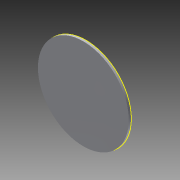
# Autodesk Inventor part: basis
Saved by Autodesk Inventor 2014 (Build 180170000, 170)
## iProperties
Created: 2015-03-19
Part Number: basis
Material: ABS Plastic
Document SubType Name: Modeling
Designer: MSI
Density: 1 g/cm^3
Appearance: Smooth - White
Author: MSI
Autodesk Inventor part; units mm, degrees
ref_plane "YZ Plane" through (0, 0, 0) normal (1, 0, 0) x (0, 1, 0)
ref_plane "XZ Plane" through (0, 0, 0) normal (0, 1, 0) x (-1, 0, 0)
ref_plane "XY Plane" through (0, 0, 0) normal (0, 0, 1) x (1, 0, 0)
sketch "Sketch1" plane through (0, 0, 0) normal (0, 1, 0) x (-1, 0, 0)
  circle A0 centre (0, 0) radius 77.5
  dimension "d0" = 155
  constraints: 1 centre point, 1 coincident
  measures "d0" diameter of A0
extrude "Extrusion1" add sketch "Sketch1" along normal blind 2
sketch "Sketch2" plane through (0, 2, 0) normal (0, 1, 0) x (1, 0, 0)
  circle A0 centre (0, 0) radius 77.5 projected
  line L0 (0, 0) -> (0, 77.5) construction
  line L1 (0, 0) -> (3.3805, 77.4262) construction
  line L2 (0, 0) -> (-3.3805, 77.4262) construction
  line L3 (0, 0) -> (-67.117, 38.75) construction
  line L4 (0, 0) -> (-65.3628, 41.6407) construction
  line L5 (0, 0) -> (-68.7433, 35.7855) construction
  line L6 (0, 0) -> (-67.117, -38.75) construction
  line L7 (0, 0) -> (-68.7433, -35.7855) construction
  line L8 (0, 0) -> (-65.3628, -41.6407) construction
  line L9 (0, 0) -> (0, -77.5) construction
  line L10 (0, 0) -> (-3.3805, -77.4262) construction
  line L11 (0, 0) -> (3.3805, -77.4262) construction
  line L12 (0, 0) -> (67.117, -38.75) construction
  line L13 (0, 0) -> (65.3628, -41.6407) construction
  line L14 (0, 0) -> (68.7433, -35.7855) construction
  line L15 (0, 0) -> (67.117, 38.75) construction
  line L16 (0, 0) -> (68.7433, 35.7855) construction
  line L17 (0, 0) -> (65.3628, 41.6407) construction
  arc A1 (46.2658, -18.96) -> (46.2658, 18.96) centre (0, 0) ccw
  arc A2 (6.7131, -49.5473) -> (39.5527, -30.5873) centre (0, 0) ccw
  arc A3 (-39.5527, -30.5873) -> (-6.7131, -49.5473) centre (0, 0) ccw
  arc A4 (-46.2658, 18.96) -> (-46.2658, -18.96) centre (0, 0) ccw
  arc A5 (-6.7131, 49.5473) -> (-39.5527, 30.5873) centre (0, 0) ccw
  arc A6 (39.5527, 30.5873) -> (6.7131, 49.5473) centre (0, 0) ccw
  arc A7 (55.9693, 42.0409) -> (8.4238, 69.4913) centre (0, 0) ccw
  arc A8 (64.3931, -27.4504) -> (64.3931, 27.4504) centre (0, 0) ccw
  arc A9 (8.4238, -69.4913) -> (55.9693, -42.0409) centre (0, 0) ccw
  arc A10 (-55.9693, -42.0409) -> (-8.4238, -69.4913) centre (0, 0) ccw
  arc A11 (-64.3931, 27.4504) -> (-64.3931, -27.4504) centre (0, 0) ccw
  arc A12 (-8.4238, 69.4913) -> (-55.9693, 42.0409) centre (0, 0) ccw
  line L18 (-2.3891, 54.7201) -> (-2.8269, 64.7457)
  line L19 (-46.1945, 29.4291) -> (-54.658, 34.821)
  line L20 (2.3891, 54.7201) -> (2.8269, 64.7457)
  line L21 (46.1945, 29.4291) -> (54.658, 34.821)
  line L22 (48.5836, 25.291) -> (57.4849, 29.9247)
  line L23 (48.5836, -25.291) -> (57.4849, -29.9247)
  line L24 (46.1945, -29.4291) -> (54.658, -34.821)
  line L25 (2.3891, -54.7201) -> (2.8269, -64.7457)
  line L26 (-2.3891, -54.7201) -> (-2.8269, -64.7457)
  line L27 (-46.1945, -29.4291) -> (-54.658, -34.821)
  line L28 (-48.5836, -25.291) -> (-57.4849, -29.9247)
  line L29 (-48.5836, 25.291) -> (-57.4849, 29.9247)
  arc A13 (-46.1945, 29.4291) -> (-39.5527, 30.5873) centre (-43.508, 33.6461) ccw
  arc A14 (-6.7131, 49.5473) -> (-2.3891, 54.7201) centre (-7.3844, 54.502) ccw
  arc A15 (-2.8269, 64.7457) -> (-8.4238, 69.4913) centre (-7.8221, 64.5276) ccw
  arc A16 (-55.9693, 42.0409) -> (-54.658, 34.821) centre (-51.9715, 39.038) ccw
  arc A17 (2.3891, 54.7201) -> (6.7131, 49.5473) centre (7.3844, 54.502) ccw
  arc A18 (8.4238, 69.4913) -> (2.8269, 64.7457) centre (7.8221, 64.5276) ccw
  arc A19 (54.658, 34.821) -> (55.9693, 42.0409) centre (51.9715, 39.038) ccw
  arc A20 (39.5527, 30.5873) -> (46.1945, 29.4291) centre (43.508, 33.6461) ccw
  arc A21 (48.5836, 25.291) -> (46.2658, 18.96) centre (50.8923, 20.856) ccw
  arc A22 (46.2658, -18.96) -> (48.5836, -25.291) centre (50.8923, -20.856) ccw
  arc A23 (57.4849, -29.9247) -> (64.3931, -27.4504) centre (59.7936, -25.4897) ccw
  arc A24 (64.3931, 27.4504) -> (57.4849, 29.9247) centre (59.7936, 25.4897) ccw
  arc A25 (46.1945, -29.4291) -> (39.5527, -30.5873) centre (43.508, -33.6461) ccw
  arc A26 (6.7131, -49.5473) -> (2.3891, -54.7201) centre (7.3844, -54.502) ccw
  arc A27 (2.8269, -64.7457) -> (8.4238, -69.4913) centre (7.8221, -64.5276) ccw
  arc A28 (55.9693, -42.0409) -> (54.658, -34.821) centre (51.9715, -39.038) ccw
  arc A29 (-2.3891, -54.7201) -> (-6.7131, -49.5473) centre (-7.3844, -54.502) ccw
  arc A30 (-8.4238, -69.4913) -> (-2.8269, -64.7457) centre (-7.8221, -64.5276) ccw
  arc A31 (-54.658, -34.821) -> (-55.9693, -42.0409) centre (-51.9715, -39.038) ccw
  arc A32 (-39.5527, -30.5873) -> (-46.1945, -29.4291) centre (-43.508, -33.6461) ccw
  arc A33 (-48.5836, -25.291) -> (-46.2658, -18.96) centre (-50.8923, -20.856) ccw
  arc A34 (-46.2658, 18.96) -> (-48.5836, 25.291) centre (-50.8923, 20.856) ccw
  arc A35 (-57.4849, 29.9247) -> (-64.3931, 27.4504) centre (-59.7936, 25.4897) ccw
  arc A36 (-64.3931, -27.4504) -> (-57.4849, -29.9247) centre (-59.7936, -25.4897) ccw
  point P0 (44.3505, -23.0874)
  point P1 (44.3505, 23.0874)
  point P2 (42.1696, -26.865)
  point P3 (2.181, -49.9524)
  point P4 (-2.181, -49.9524)
  point P5 (-42.1696, -26.865)
  point P6 (-44.3505, -23.0874)
  point P7 (-44.3505, 23.0874)
  point P8 (-42.1696, 26.865)
  point P9 (-2.181, 49.9524)
  point P10 (2.181, 49.9524)
  point P11 (42.1696, 26.865)
  point P12 (59.0374, 37.611)
  point P13 (3.0534, 69.9334)
  point P14 (62.0908, 32.3224)
  point P15 (62.0908, -32.3224)
  point P16 (59.0374, -37.611)
  point P17 (3.0534, -69.9334)
  point P18 (-3.0534, -69.9334)
  point P19 (-59.0374, -37.611)
  point P20 (-62.0908, -32.3224)
  point P21 (-62.0908, 32.3224)
  point P22 (-59.0374, 37.611)
  point P23 (-3.0534, 69.9334)
  dimension "d15" = 2.5
  dimension "d18" = 360
  dimension "d21" = 50
  dimension "d22" = 50
  dimension "d23" = 50
  dimension "d24" = 50
  dimension "d25" = 50
  dimension "d26" = 50
  dimension "d28" = 70
  dimension "d29" = 70
  dimension "d30" = 70
  dimension "d31" = 70
  dimension "d32" = 70
  dimension "d33" = 70
  dimension "d34" = 5
  constraints: 98 point on circle, 60 end point, 48 point on line, 48 tangent, 36 centre point, 23 equal radius, 12 collinear, 4 coincident, 1 symmetric about line, 1 vertical alignment, 41 other
  measures "d15" angle of L0 L1
  measures "d21" radius of A5
  measures "d22" radius of A6
  measures "d23" radius of A1
  measures "d24" radius of A2
  measures "d25" radius of A3
  measures "d26" radius of A4
  measures "d28" radius of A7
  measures "d29" radius of A8
  measures "d30" radius of A9
  measures "d31" radius of A10
  measures "d32" radius of A11
  measures "d33" radius of A12
  measures "d34" radius of A13
extrude "Extrusion2" add sketch "Sketch2" along normal blind 2
sketch "Sketch3" plane through (0, 4, 0) normal (0, 1, 0) x (1, 0, 0)
  circle A0 centre (0, 0) radius 77.5 projected
  circle A1 centre (0, 0) radius 6.4
  dimension "d37" = 12.8
  constraints: 1 centre point, 1 coincident
  measures "d37" diameter of A1
extrude "Extrusion3" add sketch "Sketch3" along normal blind 6.6 contours A1
sketch "Sketch4" plane through (0, 10.6, 0) normal (0, 1, 0) x (1, 0, 0)
  circle A0 centre (0, 0) radius 6.4 projected
  circle A1 centre (0, 0) radius 2.2
  dimension "d40" = 4.4
  constraints: 1 centre point, 1 coincident
  measures "d40" diameter of A1
extrude "Extrusion4" add sketch "Sketch4" along normal blind 12 contours A1
fillet "Fillet1" radius 5 1 edges at (-6.4, 4, 0)
sketch "Sketch5" plane through (0, 4, 0) normal (0, 1, 0) x (1, 0, 0)
  circle A0 centre (0, 0) radius 77.5 projected
  line L0 (-48.5836, -25.291) -> (-57.4849, -29.9247) projected
  arc A1 (-64.3931, -27.4504) -> (-57.4849, -29.9247) centre (-59.7936, -25.4897) ccw projected
  arc A2 (-64.3931, 27.4504) -> (-64.3931, -27.4504) centre (0, 0) ccw projected
  arc A3 (-57.4849, 29.9247) -> (-64.3931, 27.4504) centre (-59.7936, 25.4897) ccw projected
  line L1 (-57.4849, 29.9247) -> (-48.5836, 25.291) projected
  arc A4 (-46.2658, 18.96) -> (-48.5836, 25.291) centre (-50.8923, 20.856) ccw projected
  arc A5 (-46.2658, 18.96) -> (-46.2658, -18.96) centre (0, 0) ccw projected
  arc A6 (-48.5836, -25.291) -> (-46.2658, -18.96) centre (-50.8923, -20.856) ccw projected
  line L2 (-46.1945, 29.4291) -> (-54.658, 34.821) projected
  arc A7 (-55.9693, 42.0409) -> (-54.658, 34.821) centre (-51.9715, 39.038) ccw projected
  arc A8 (-8.4238, 69.4913) -> (-55.9693, 42.0409) centre (0, 0) ccw projected
  arc A9 (-2.8269, 64.7457) -> (-8.4238, 69.4913) centre (-7.8221, 64.5276) ccw projected
  line L3 (-2.8269, 64.7457) -> (-2.3891, 54.7201) projected
  arc A10 (-6.7131, 49.5473) -> (-2.3891, 54.7201) centre (-7.3844, 54.502) ccw projected
  arc A11 (-6.7131, 49.5473) -> (-39.5527, 30.5873) centre (0, 0) ccw projected
  arc A12 (-46.1945, 29.4291) -> (-39.5527, 30.5873) centre (-43.508, 33.6461) ccw projected
  line L4 (46.1945, -29.4291) -> (54.658, -34.821) projected
  arc A13 (55.9693, -42.0409) -> (54.658, -34.821) centre (51.9715, -39.038) ccw projected
  arc A14 (8.4238, -69.4913) -> (55.9693, -42.0409) centre (0, 0) ccw projected
  arc A15 (2.8269, -64.7457) -> (8.4238, -69.4913) centre (7.8221, -64.5276) ccw projected
  line L5 (2.8269, -64.7457) -> (2.3891, -54.7201) projected
  arc A16 (6.7131, -49.5473) -> (2.3891, -54.7201) centre (7.3844, -54.502) ccw projected
  arc A17 (6.7131, -49.5473) -> (39.5527, -30.5873) centre (0, 0) ccw projected
  arc A18 (46.1945, -29.4291) -> (39.5527, -30.5873) centre (43.508, -33.6461) ccw projected
  line L6 (48.5836, 25.291) -> (57.4849, 29.9247) projected
  arc A19 (64.3931, 27.4504) -> (57.4849, 29.9247) centre (59.7936, 25.4897) ccw projected
  arc A20 (64.3931, -27.4504) -> (64.3931, 27.4504) centre (0, 0) ccw projected
  arc A21 (57.4849, -29.9247) -> (64.3931, -27.4504) centre (59.7936, -25.4897) ccw projected
  line L7 (57.4849, -29.9247) -> (48.5836, -25.291) projected
  arc A22 (46.2658, -18.96) -> (48.5836, -25.291) centre (50.8923, -20.856) ccw projected
  arc A23 (46.2658, -18.96) -> (46.2658, 18.96) centre (0, 0) ccw projected
  arc A24 (48.5836, 25.291) -> (46.2658, 18.96) centre (50.8923, 20.856) ccw projected
  line L8 (2.3891, 54.7201) -> (2.8269, 64.7457) projected
  arc A25 (8.4238, 69.4913) -> (2.8269, 64.7457) centre (7.8221, 64.5276) ccw projected
  arc A26 (55.9693, 42.0409) -> (8.4238, 69.4913) centre (0, 0) ccw projected
  arc A27 (54.658, 34.821) -> (55.9693, 42.0409) centre (51.9715, 39.038) ccw projected
  line L9 (54.658, 34.821) -> (46.1945, 29.4291) projected
  arc A28 (39.5527, 30.5873) -> (46.1945, 29.4291) centre (43.508, 33.6461) ccw projected
  arc A29 (39.5527, 30.5873) -> (6.7131, 49.5473) centre (0, 0) ccw projected
  arc A30 (2.3891, 54.7201) -> (6.7131, 49.5473) centre (7.3844, 54.502) ccw projected
  line L10 (-2.3891, -54.7201) -> (-2.8269, -64.7457) projected
  arc A31 (-8.4238, -69.4913) -> (-2.8269, -64.7457) centre (-7.8221, -64.5276) ccw projected
  arc A32 (-55.9693, -42.0409) -> (-8.4238, -69.4913) centre (0, 0) ccw projected
  arc A33 (-54.658, -34.821) -> (-55.9693, -42.0409) centre (-51.9715, -39.038) ccw projected
  line L11 (-54.658, -34.821) -> (-46.1945, -29.4291) projected
  arc A34 (-39.5527, -30.5873) -> (-46.1945, -29.4291) centre (-43.508, -33.6461) ccw projected
  arc A35 (-39.5527, -30.5873) -> (-6.7131, -49.5473) centre (0, 0) ccw projected
  arc A36 (-2.3891, -54.7201) -> (-6.7131, -49.5473) centre (-7.3844, -54.502) ccw projected
  circle A37 centre (0, 0) radius 11.4 projected
sketch "Sketch6" plane through (0, 4, 0) normal (0, 1, 0) x (1, 0, 0)
  circle A0 centre (0, 0) radius 11.4 projected
  circle A1 centre (0, 0) radius 39.5
  circle A2 centre (0, 0) radius 37.5
  dimension "d44" = 79
  dimension "d45" = 75
  constraints: 2 centre point, 2 coincident
  measures "d44" diameter of A1
  measures "d45" diameter of A2
extrude "Extrusion5" cut sketch "Sketch6" against normal blind 1 contours A1
body "Solid1"
